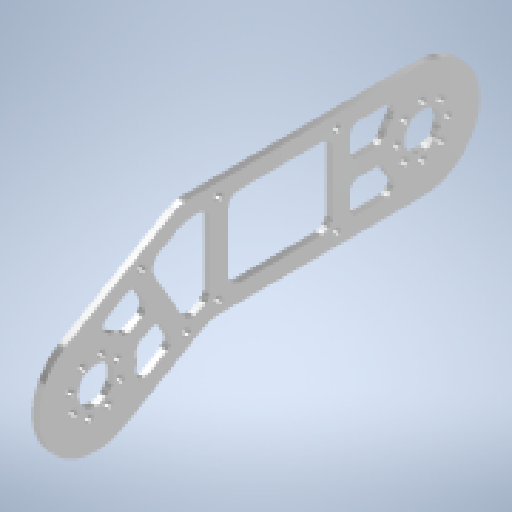
# Autodesk Inventor part: leg_upper
Saved by Autodesk Inventor 2024.1 (Build 281209000, 209)
## iProperties
Created: 2023-08-04
Part Number: leg_upper
Material: アルミニウム 6061
Document SubType Name: Modeling
Designer: hibik
Density: 2.7 g/cm^3
Appearance: アルミニウム - フラット
Author: hibik
Autodesk Inventor part; units mm, degrees
ref_plane "YZ Plane" through (0, 0, 0) normal (1, 0, 0) x (0, 1, 0)
ref_plane "XZ Plane" through (0, 0, 0) normal (0, 1, 0) x (-1, 0, 0)
ref_plane "XY Plane" through (0, 0, 0) normal (0, 0, 1) x (1, 0, 0)
sketch "スケッチ1" plane through (0, 0, 0) normal (1, 0, 0) x (0, 1, 0)
  line L0 (27, 0) -> (0, 0)
  line L1 (0, 0) -> (0, -65.872265)
  line L2 (0, -65.872265) -> (27, -65.872265)
  line L3 (27, -65.872265) -> (27, 0)
  line L4 (27, 0) -> (7.296343, 34.127735)
  line L5 (7.296343, 34.127735) -> (-16.086343, 20.627735)
  line L6 (-16.086343, 20.627735) -> (0, -7.234628)
  line L7 (0, 19.765372) -> (-4.395, 27.377735)
  circle A0 centre (0, 19.765372) radius 4.25
  circle A1 centre (13.5, -57.082265) radius 4.25
  line L8 (13.5, -65.872265) -> (13.5, -57.082265)
  circle A2 centre (0, 19.765372) radius 13.5
  circle A3 centre (13.5, -57.082265) radius 13.5
  line L9 (5.064542, 0) -> (22.68082, 0)
  circle A4 centre (0, 19.765372) radius 6
  circle A5 centre (13.5, -57.082265) radius 6
  circle A6 centre (-3, 24.961524) radius 1
  circle A7 centre (-5.795555, 21.318286) radius 1
  circle A8 centre (-5.196152, 16.765372) radius 1
  circle A9 centre (-1.552914, 13.969817) radius 1
  circle A10 centre (3, 14.569219) radius 1
  circle A11 centre (5.795555, 18.212458) radius 1
  circle A12 centre (13.5, -63.082265) radius 1
  circle A13 centre (17.742641, -61.324906) radius 1
  circle A14 centre (19.5, -57.082265) radius 1
  circle A15 centre (17.742641, -52.839624) radius 1
  circle A16 centre (13.5, -51.082265) radius 1
  circle A17 centre (9.257359, -52.839624) radius 1
  circle A18 centre (7.5, -57.082265) radius 1
  circle A19 centre (9.257359, -61.324906) radius 1
  circle A20 centre (5.196152, 22.765372) radius 1
  circle A21 centre (1.552914, 25.560927) radius 1
  point P0 (-11.691343, 13.015372)
  point P1 (0, -57.082265)
  point P2 (27, -57.082265)
  point P3 (11.691343, 26.515372)
  dimension "d79" = 12
  dimension "d80" = 12
  dimension "d0" = 27
  dimension "d10" = 150
  dimension "d11" = 27
  dimension "d13" = 8.79
  dimension "d14" = 100
  dimension "d15" = 8.79
  dimension "d16" = 8.5
  dimension "d81" = 2
  dimension "d84" = 360
  dimension "d86" = 2
  dimension "d89" = 360
  dimension "d100" = 39.40731
  constraints: 20 centre point, 20 end point, 7 coincident, 4 point on line, 3 perpendicular, 2 midpoint, 2 parallel, 2 tangent, 2 vertical alignment, 1 equal radius, 1 horizontal, 1 vertical, 40 other
  measures "d0" distance of L1.end L2.end
  measures "d10" angle of L3 L4
  measures "d11" distance between parallel lines of L6 L4
  measures "d13" distance from line of L5 L7.start
  measures "d14" distance from line of L2 L4.end
  measures "d15" distance of L8.start point (13.5, -57.082)
  measures "d16" diameter of A0
  measures "d81" diameter of A6
  measures "d86" diameter of A12
  measures "d100" distance from line of L0.start L5
sketch "スケッチ1 outline for 押し出し1" plane through (0, 0, 0) normal (1, 0, 0) x (0, 1, 0)
  arc A0 (11.691343, 26.515372) -> (-11.691343, 13.015372) centre (0, 19.765372) ccw
  line L0 (27, 0) -> (11.691343, 26.515372)
  line L1 (-11.691343, 13.015372) -> (0, -7.234628)
  line L2 (27, -57.082265) -> (27, 0)
  line L3 (0, -7.234628) -> (0, -57.082265)
  arc A1 (0, -57.082265) -> (27, -57.082265) centre (13.5, -57.082265) ccw
  circle A2 centre (9.257359, -61.324906) radius 1
  circle A3 centre (7.5, -57.082265) radius 1
  circle A4 centre (9.257359, -52.839624) radius 1
  circle A5 centre (13.5, -63.082265) radius 1
  circle A6 centre (13.5, -57.082265) radius 4.25
  circle A7 centre (13.5, -51.082265) radius 1
  circle A8 centre (17.742641, -61.324906) radius 1
  circle A9 centre (17.742641, -52.839624) radius 1
  circle A10 centre (19.5, -57.082265) radius 1
  circle A11 centre (-1.552914, 13.969817) radius 1
  circle A12 centre (-5.196152, 16.765372) radius 1
  circle A13 centre (-5.795555, 21.318286) radius 1
  circle A14 centre (0, 19.765372) radius 4.25
  circle A15 centre (-3, 24.961524) radius 1
  circle A16 centre (3, 14.569219) radius 1
  circle A17 centre (1.552914, 25.560927) radius 1
  circle A18 centre (5.795555, 18.212458) radius 1
  circle A19 centre (5.196152, 22.765372) radius 1
extrude "押し出し1" add sketch "スケッチ1 outline for 押し出し1" along normal blind 1.5
fillet "フィレット1" radius 8 2 edges at (0.75, 27, 0) (0.75, 0, -7.2346)
sketch "スケッチ8 outline for 押し出し9" plane through (1.5, 0, 0) normal (1, 0, 0) x (0, 0, -1)
  circle A0 centre (-8.892305, 18.401924) radius 1
  circle A1 centre (9.234628, 3) radius 1
  circle A2 centre (9.234628, 24) radius 1
  circle A3 centre (37, 3) radius 1
  circle A4 centre (37, 24) radius 1
  circle A5 centre (1.607695, 0.21539) radius 1
  arc A6 (33, 4) -> (36, 7) centre (33, 7) ccw
  line L0 (14.234628, 4) -> (33, 4)
  arc A7 (11.234628, 7) -> (14.234628, 4) centre (14.234628, 7) ccw
  line L1 (11.234628, 20) -> (11.234628, 7)
  arc A8 (14.234628, 23) -> (11.234628, 20) centre (14.234628, 20) ccw
  line L2 (33, 23) -> (14.234628, 23)
  arc A9 (36, 20) -> (33, 23) centre (33, 20) ccw
  line L3 (36, 7) -> (36, 20)
  arc A10 (3.21539, 23) -> (-0.78461, 21.928203) centre (3.21539, 15) ccw
  line L4 (4.234628, 23) -> (3.21539, 23)
  arc A11 (7.234628, 20) -> (4.234628, 23) centre (4.234628, 20) ccw
  line L5 (7.234628, 6.221497) -> (7.234628, 20)
  arc A12 (5.349506, 3.436349) -> (7.234628, 6.221497) centre (4.234628, 6.221497) ccw
  arc A13 (4.50518, 3.039791) -> (5.349506, 3.436349) centre (8.322513, -3.990712) cw
  arc A14 (0.475604, 4.17623) -> (4.50518, 3.039791) centre (3.07368, 5.67623) ccw
  line L6 (-6.026279, 15.437822) -> (0.475604, 4.17623)
  arc A15 (-4.928203, 19.535898) -> (-6.026279, 15.437822) centre (-3.428203, 16.937822) ccw
  line L7 (-0.78461, 21.928203) -> (-4.928203, 19.535898)
  line L8 (47.795177, 11.5) -> (40, 11.5)
  arc A16 (57.082265, 4) -> (47.795177, 11.5) centre (57.082265, 13.5) cw
  line L9 (40, 4) -> (57.082265, 4)
  line L10 (40, 11.5) -> (40, 4)
  line L11 (40, 15.5) -> (47.795177, 15.5)
  line L12 (40, 23) -> (40, 15.5)
  line L13 (57.082265, 23) -> (40, 23)
  arc A17 (47.795177, 15.5) -> (57.082265, 23) centre (57.082265, 13.5) cw
  line L14 (-5.240381, 6.076606) -> (-10.722518, 2.911493)
  line L15 (-1.490381, -0.418584) -> (-5.240381, 6.076606)
  line L16 (-15.015372, -8.227241) -> (-1.490381, -0.418584)
  arc A18 (-10.722518, 2.911493) -> (-15.015372, -8.227241) centre (-19.765372, 0) cw
  line L17 (-12.722518, 6.375595) -> (-7.240381, 9.540708)
  arc A19 (-24.515372, 8.227241) -> (-12.722518, 6.375595) centre (-19.765372, 0) cw
  line L18 (-10.990381, 16.035898) -> (-24.515372, 8.227241)
  line L19 (-7.240381, 9.540708) -> (-10.990381, 16.035898)
extrude "押し出し9" cut sketch "スケッチ8 outline for 押し出し9" against normal through all
fillet "フィレット4" radius 2 16 edges at (0.75, 8.2272, 24.5154) (0.75, -8.2272, 15.0154) (0.75, -0.4186, 1.4904) (0.75, 6.0766, 5.2404) (0.75, 2.9115, 10.7225) (0.75, 6.3756, 12.7225) (0.75, 9.5407, 7.2404) (0.75, 16.0359, 10.9904) (0.75, 4, -40) (0.75, 11.5, -40) (0.75, 23, -40) (0.75, 15.5, -40) (0.75, 23, -57.0823) (0.75, 15.5, -47.7952) (0.75, 11.5, -47.7952) (0.75, 4, -57.0823)
equation "\"d97\" = d95"
equation "\"d98\" = d96"
equation "\"d95\" = 4"
equation "\"d96\" = 4"
